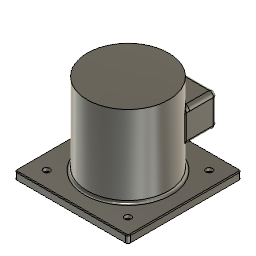
Base (Autodesk Fusion 360 design; units mm, degrees)
part number: 2026-08-18-15-37-16-751
Autodesk Fusion 360 part; units mm, degrees
sketch "Sketch1" plane through (0, 0, 0) normal (0, 0, 1) x (1, 0, 0)
  line L0 (70, 70) -> (-70, 70)
  line L1 (-70, 70) -> (-70, -70)
  line L2 (-70, -70) -> (70, -70)
  line L3 (70, -70) -> (70, 70)
  line L4 (70, 70) -> (-70, -70) construction
  line L5 (-70, 70) -> (70, -70) construction
  dimension "d1" = 140
  dimension "d2" = 140
  constraint horizontal L0
  constraint perpendicular L0 L1
  constraint parallel L0 L2
  constraint parallel L1 L3
  constraint coincident L4 origin
  constraint coincident L5 origin
  measures "d1" distance of L1.end L2.end
  measures "d2" distance of L0.end L1.end
extrude "Extrude1" add sketch "Sketch1" along normal blind 10
sketch "Sketch2" plane through (0, 0, 10) normal (0, 0, 1) x (-1, 0, 0)
  line L0 (-70, 70) -> (-70, -70)
  line L1 (-70, -70) -> (70, -70)
  line L2 (70, -70) -> (70, 70)
  line L3 (70, 70) -> (-70, 70)
  circle A0 centre (0, 0) radius 50
  dimension "d5" = 100
  constraint coincident A0.centre origin
  measures "d5" diameter of A0
extrude "Extrude2" add sketch "Sketch2" along normal blind 100 contours A0
sketch "Sketch3" plane through (0, 0, 0) normal (0, 1, 0) x (1, 0, 0)
  line L0 (-40, -80) -> (40, -80)
  line L1 (40, -80) -> (40, -40)
  line L2 (40, -40) -> (-40, -40)
  line L3 (-40, -40) -> (-40, -80)
  dimension "d8" = 80
  dimension "d9" = 40
  dimension "d10" = 40
  dimension "d11" = 40
  constraint horizontal L0
  constraint vertical L1
  constraint horizontal L2
  constraint vertical L3
  measures "d8" distance of L0.start L0.end
  measures "d9" distance of L0.start L2.end
  measures "d10" vertical distance of origin L2.end
  measures "d11" distance of origin L1
extrude "Extrude3" add sketch "Sketch3" along normal blind 70
sketch "Sketch4" plane through (0, 0, 110) normal (0, 0, 1) x (-1, 0, 0)
  circle A0 centre (0, 0) radius 50
  circle A1 centre (0, 0) radius 47.5
  dimension "d14" = 95
  constraint coincident A0.centre A1.centre
  measures "d14" diameter of A1
sketch "Sketch6" plane through (0, 0, 10) normal (0, 0, 1) x (-1, 0, 0)
  circle A0 centre (0, 0) radius 50
  line L0 (-70, 70) -> (-70, -70)
  line L1 (-70, -70) -> (70, -70)
  line L2 (70, -70) -> (70, 70)
  line L3 (70, 70) -> (-70, 70)
  point P0 (-50, 50)
  point P1 (50, 50)
  point P2 (50, -50)
  point P3 (-50, -50)
  dimension "d17" = 20
  dimension "d18" = 20
  dimension "d19" = 20
  dimension "d20" = 20
  dimension "d21" = 20
  dimension "d22" = 20
  dimension "d23" = 20
  dimension "d24" = 20
  measures "d17" distance of L0 P0
  measures "d18" distance of L3 P0
  measures "d19" distance of L3 P1
  measures "d20" distance of L2 P1
  measures "d21" distance of L2 P2
  measures "d22" distance of L1 P2
  measures "d23" distance of L1 P3
  measures "d24" distance of L0 P3
hole "Hole1" at (50, -50, 10) at (50, 50, 10) at (-50, 50, 10) at (-50, -50, 10) direction (0, 0, -1) diameter 4.5 depth 20 tip angle 118 counterbore diameter 8 counterbore depth 4
fillet "Fillet1" radius 3 4 edges at (-70, 70, 5) (70, 70, 5) (70, -70, 5) (-70, -70, 5)
fillet "Fillet2" radius 5 6 edges at (0, 70, 80) (0, 70, 40) (-40, 70, 60) (40, 70, 60) (-40, 30, 60) (40, 30, 60)
fillet "Fillet3" radius 3 1 edges at (46.6164, -18.0808, 10)
fillet "Fillet4" radius 1 16 edges at (-69.1213, -69.1213, 10) (0, -70, 10) (69.1213, -69.1213, 10) (70, 0, 10) (69.1213, 69.1213, 10) (0, 70, 10) (-69.1213, 69.1213, 10) (-70, 0, 10) (0, -70, 0) (69.1213, -69.1213, 0) (70, 0, 0) (69.1213, 69.1213, 0) (0, 70, 0) (-69.1213, 69.1213, 0) (-70, 0, 0) (-69.1213, -69.1213, 0)
fillet "Fillet5" radius 5 12 edges at (-40.2327, 30.1152, 80) (-40, 48.3114, 80) (-38.5355, 68.5355, 78.5355) (-40.2327, 30.1152, 40) (-40, 48.3114, 40) (-38.5355, 68.5355, 41.4645) (40.2327, 30.1152, 80) (40, 48.3114, 80) (38.5355, 68.5355, 78.5355) (40.2327, 30.1152, 40) (40, 48.3114, 40) (38.5355, 68.5355, 41.4645)
